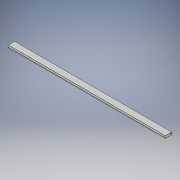
# Autodesk Inventor part: the smaller outside for the 2nd slider part
Saved by Autodesk Inventor 2017 (Build 210142000, 142)
## iProperties
Created: 2019-02-04
Part Number: the smaller outside for the 2nd slider part
Material: Generic
Document SubType Name: Modeling
Designer: S346852600
Density: 1 g/cm^3
Appearance: Default
Author: S346852600
Autodesk Inventor part; units mm, degrees
ref_plane "YZ Plane" through (0, 0, 0) normal (1, 0, 0) x (0, 1, 0)
ref_plane "XZ Plane" through (0, 0, 0) normal (0, 1, 0) x (-1, 0, 0)
ref_plane "XY Plane" through (0, 0, 0) normal (0, 0, 1) x (1, 0, 0)
sketch "Sketch1" plane through (0, 0, 0) normal (1, 0, 0) x (0, 1, 0)
  line L0 (0, -0.4446) -> (0, -24.9554)
  line L1 (-0.4178, -25.5521) -> (-4.3558, -26.9854)
  line L2 (-0.4178, 0.1521) -> (-4.3558, 1.5854)
  line L3 (-5.0594, 1.3969) -> (-6.4063, -0.2083)
  line L4 (-4.8497, -23.8856) -> (-4.8389, -24.1212)
  line L5 (-3.9874, -24.6889) -> (-2.4498, -24.1293)
  line L6 (-2.032, -23.5325) -> (-2.032, -1.8675)
  line L7 (-2.4498, -1.2707) -> (-3.7138, -0.8107)
  line L8 (-4.4174, -0.9992) -> (-4.8497, -1.5144)
  line L9 (-6.4063, -0.2083) -> (-4.8497, -1.5144)
  arc A0 (0, -0.4446) -> (-0.4178, 0.1521) centre (-0.635, -0.4446) ccw
  arc A1 (-2.032, -1.8675) -> (-2.4498, -1.2707) centre (-2.667, -1.8675) ccw
  arc A2 (-4.3558, 1.5854) -> (-5.0594, 1.3969) centre (-4.573, 0.9887) ccw
  arc A3 (-3.7138, -0.8107) -> (-4.4174, -0.9992) centre (-3.931, -1.4074) ccw
  arc A4 (-2.4498, -24.1293) -> (-2.032, -23.5325) centre (-2.667, -23.5325) ccw
  arc A5 (-0.4178, -25.5521) -> (0, -24.9554) centre (-0.635, -24.9554) ccw
  arc A6 (-4.8389, -24.1212) -> (-3.9874, -24.6889) centre (-4.2046, -24.0922) ccw
  line L10 (-4.8497, -23.8856) -> (-4.8497, -1.5144)
  line L11 (-9.6994, -0.4446) -> (-9.6994, -24.9554)
  line L12 (-9.2816, -25.5521) -> (-5.3436, -26.9854)
  line L13 (-9.2816, 0.1521) -> (-5.3436, 1.5854)
  line L14 (-4.64, 1.3969) -> (-3.2931, -0.2083)
  line L15 (-5.712, -24.6889) -> (-7.2496, -24.1293)
  line L16 (-7.6674, -23.5325) -> (-7.6674, -1.8675)
  line L17 (-7.2496, -1.2707) -> (-5.9856, -0.8107)
  line L18 (-5.282, -0.9992) -> (-4.8497, -1.5144)
  line L19 (-3.2931, -0.2083) -> (-4.8497, -1.5144)
  arc A7 (-9.2816, 0.1521) -> (-9.6994, -0.4446) centre (-9.0644, -0.4446) ccw
  arc A8 (-7.2496, -1.2707) -> (-7.6674, -1.8675) centre (-7.0324, -1.8675) ccw
  arc A9 (-4.64, 1.3969) -> (-5.3436, 1.5854) centre (-5.1264, 0.9887) ccw
  arc A10 (-5.282, -0.9992) -> (-5.9856, -0.8107) centre (-5.7685, -1.4074) ccw
  arc A11 (-7.6674, -23.5325) -> (-7.2496, -24.1293) centre (-7.0324, -23.5325) ccw
  arc A12 (-9.6994, -24.9554) -> (-9.2816, -25.5521) centre (-9.0644, -24.9554) ccw
  arc A13 (-5.712, -24.6889) -> (-4.8605, -24.1212) centre (-5.4948, -24.0922) ccw
  line L20 (-5.3436, -26.9854) -> (-4.3558, -26.9854)
  line L21 (0, -12.7) -> (-9.6994, -12.7)
  line L22 (-5.0594, -26.7969) -> (-6.4063, -25.1917)
  line L23 (-4.8389, -24.1212) -> (-4.8497, -23.8856)
  line L24 (-6.4063, -25.1917) -> (-4.8497, -23.8856)
  arc A14 (-5.0594, -26.7969) -> (-4.3558, -26.9854) centre (-4.573, -26.3887) ccw
  arc A15 (-5.3436, -26.9854) -> (-4.64, -26.7969) centre (-5.1264, -26.3887) ccw
  line L25 (-4.64, -26.7969) -> (-3.2931, -25.1917)
  line L26 (-4.8605, -24.1212) -> (-4.8497, -23.8856)
  line L27 (-3.2931, -25.1917) -> (-4.8497, -23.8856)
  point P0 (0, 0)
  point P1 (0, -25.4)
  point P2 (-4.7736, -27.1375)
  point P3 (-4.7736, 1.7375)
  point P4 (-4.7995, -24.9845)
  point P5 (-2.032, -23.9772)
  point P6 (-2.032, -1.4228)
  point P7 (-4.1316, -0.6586)
  dimension "d0" = 25.4
  dimension "d4" = 5.08
  dimension "d5" = 110
  dimension "d8" = 5.08
  dimension "d10" = 110
  dimension "d11" = 2.54
  dimension "d12" = 110
  dimension "d13" = 2.032
  dimension "d16" = 0.635
  dimension "d18" = 2.032
  constraints: 56 end point, 32 point on circle, 29 symmetric about line, 16 centre point, 15 point on line, 14 tangent, 6 equal radius, 2 midpoint, 1 horizontal, 1 perpendicular, 1 vertical, 12 other
  measures "d0" distance of point (0, 0) point (0, -25.4)
  measures "d4" distance of point (0, -25.4) point (-4.774, -27.137)
  measures "d5" angle of L1 L0
  measures "d8" distance of point (0, 0) point (-4.774, 1.737)
  measures "d10" angle of L2 L0
  measures "d11" distance of point (-4.774, 1.737) L3.end
  measures "d12" angle of L2 L3
  measures "d13" distance between parallel lines of L0 L6
  measures "d16" radius of A0
  measures "d18" distance of L22.end L4.start
extrude "Extrusion1" add sketch "Sketch1" along normal blind 609.6 contours L0 L21 L6 A1 L7 A3 L19 L14 A9 A2 L2 A0 | L0 A5 L1 L20 A14 A15 L25 L27 L5 A4 L6 L21 | A9 L14 L19 A3 L8 L18 A10 L9 L3 A2 | A2 L3 L9 A10 L17 A8 L16 L21 L11 A7 L13 A9 | A14 L20 | L27 L5 A6 L4 | L26 A13 L15 L24 | L4 A6 L5 L27 L25 A15 A14 L22 L24 L15 A13 L26 | L9 A10 L18 | L8 A3 L19 | L16 A11 L15 L24 L22 A14 A15 L20 L12 A12 L11 L21 | A15 L20
body "Solid1"
